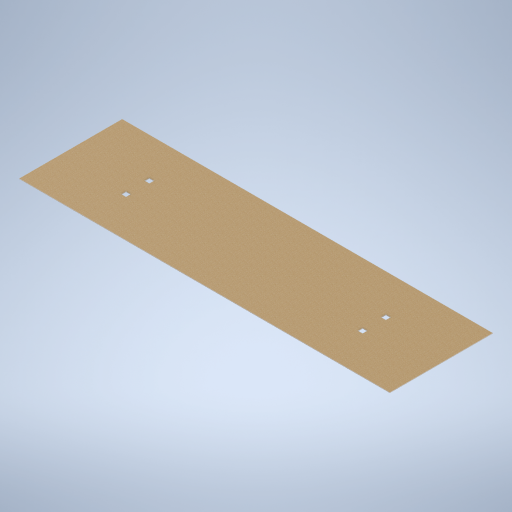
# Autodesk Inventor part: inside_floor
Saved by Autodesk Inventor 2024.2 (Build 282272000, 272)
## iProperties
Created: 2024-05-24
Part Number: inside_floor
Material: Wood (Maple)
Document SubType Name: Modeling
Designer: LOSTER_1
Density: 0.67 g/cm^3
Appearance: Natural Maple - Glossy Dark Tint
Author: LOSTER_1
Autodesk Inventor part; units mm, degrees
ref_plane "YZ Plane" through (0, 0, 0) normal (1, 0, 0) x (0, 1, 0)
ref_plane "XZ Plane" through (0, 0, 0) normal (0, 1, 0) x (-1, 0, 0)
ref_plane "XY Plane" through (0, 0, 0) normal (0, 0, 1) x (1, 0, 0)
sketch "Sketch1" plane through (0, 0, 0) normal (0, 1, 0) x (-1, 0, 0)
  line L0 (15894.0391, 4423.8081) -> (-15907.9609, 4423.8081)
  line L1 (-15907.9609, -4410.1915) -> (15894.0391, -4410.1915)
  line L2 (10343.9966, -793.1917) -> (9943.9966, -793.1917)
  line L3 (9943.9966, -793.1917) -> (9943.9966, -1193.1917)
  line L4 (9943.9966, -1193.1917) -> (10343.9966, -1193.1917)
  line L5 (10343.9966, -1193.1917) -> (10343.9966, -793.1917)
  line L6 (10343.9966, 1206.8083) -> (9943.9966, 1206.8083)
  line L7 (9943.9966, 1206.8083) -> (9943.9966, 806.8083)
  line L8 (9943.9966, 806.8083) -> (10343.9966, 806.8083)
  line L9 (10343.9966, 806.8083) -> (10343.9966, 1206.8083)
  line L10 (-9956.5806, -793.1917) -> (-10356.5806, -793.1917)
  line L11 (-10356.5806, -793.1917) -> (-10356.5806, -1193.1917)
  line L12 (-10356.5806, -1193.1917) -> (-9956.5806, -1193.1917)
  line L13 (-9956.5806, -1193.1917) -> (-9956.5806, -793.1917)
  line L14 (-9956.5806, 1206.8083) -> (-10356.5806, 1206.8083)
  line L15 (-10356.5806, 1206.8083) -> (-10356.5806, 806.8083)
  line L16 (-10356.5806, 806.8083) -> (-9956.5806, 806.8083)
  line L17 (-9956.5806, 806.8083) -> (-9956.5806, 1206.8083)
  line L18 (-15907.9609, 606.8024) -> (-14407.9609, 606.8024)
  line L19 (-14407.9609, 606.8024) -> (-14407.9609, -588.4462)
  line L20 (-14407.9609, -588.4462) -> (-15907.9609, -588.4462)
  line L21 (15894.0391, 606.8024) -> (14394.0391, 606.8024)
  line L22 (14394.0391, 606.8024) -> (14394.0391, -588.4462)
  line L23 (14394.0391, -588.4462) -> (15894.0391, -588.4462)
  line L24 (15894.0391, -4410.1915) -> (15894.0391, -588.4462)
  line L25 (15894.0391, 606.8024) -> (15894.0391, 4423.8081)
  line L26 (-15907.9609, 4423.8081) -> (-15907.9609, 606.8024)
  line L27 (-15907.9609, -588.4462) -> (-15907.9609, -4410.1915)
  point P0 (0, 0)
  point P1 (-15907.9609, -588.4462)
  point P2 (15894.0391, -588.4462)
  dimension "d0" = 1500
  dimension "d1" = 1500
  constraints: 56 end point, 11 parallel, 7 horizontal, 6 perpendicular, 1 collinear, 1 point on line, 1 vertical
  measures "d0" distance of L19.end L20.end
  measures "d1" distance of L23.end L22.end
extrude "Extrusion1" add sketch "Sketch1" along normal blind 40
sketch "Sketch2" plane through (0, 40, 0) normal (0, 1, 0) x (1, 0, 0)
  line L0 (-15894.0391, 588.4462) -> (-14394.0391, 588.4462) projected
  line L1 (-15894.0391, -606.8024) -> (-15894.0391, -4423.8081) projected
  line L2 (-15894.0391, 588.4462) -> (-15894.0391, -606.8024)
  line L3 (-15894.0391, -606.8024) -> (-14381.5011, -606.8024)
  line L4 (-14381.5011, -606.8024) -> (-14381.5011, 588.4462)
  line L5 (-14381.5011, 588.4462) -> (-15894.0391, 588.4462)
  line L6 (15907.9609, -4423.8081) -> (15907.9609, -606.8024) projected
  line L7 (14407.9609, 588.4462) -> (15907.9609, 588.4462)
  line L8 (15907.9609, 588.4462) -> (15907.9609, -606.8024)
  line L9 (15907.9609, -606.8024) -> (14407.9609, -606.8024)
  line L10 (14407.9609, -606.8024) -> (14407.9609, 588.4462)
  point P0 (0, 0)
  constraints: 16 end point, 4 perpendicular, 2 parallel, 1 horizontal, 1 vertical
extrude "Extrusion2" add sketch "Sketch2" against normal blind 40
body "Solid1"
